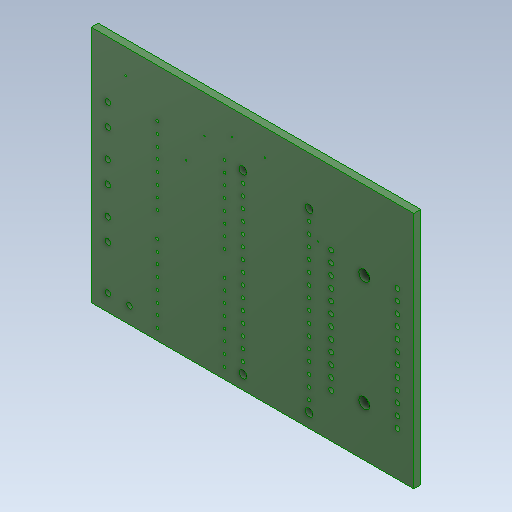
# Autodesk Inventor part: dog_driver_4.brd_Outline
Saved by Autodesk Inventor 2020 (Build 240168000, 168)
## iProperties
Created: 2019-07-14
Part Number: dog_driver_4.brd_Outline
Material: Generic
Document SubType Name: Modeling
Designer: psrob
Density: 1 g/cm^3
Appearance: Board Outline
Author: psrob
Autodesk Inventor part; units mm, degrees
ref_plane "YZ Plane" through (0, 0, 0) normal (1, 0, 0) x (0, 1, 0)
ref_plane "XZ Plane" through (0, 0, 0) normal (0, 1, 0) x (-1, 0, 0)
ref_plane "XY Plane" through (0, 0, 0) normal (0, 0, 1) x (1, 0, 0)
sketch "Sketch1" plane through (0, 0, 0) normal (0, 0, 1) x (1, 0, 0)
  line L0 (0, 0) -> (74.275, 0)
  line L1 (74.275, 0) -> (74.275, 54.915)
  line L2 (74.275, 54.915) -> (0, 54.915)
  line L3 (0, 54.915) -> (0, 0)
  circle A0 centre (50.16, 5.71) radius 0.4
  circle A1 centre (50.16, 8.26) radius 0.4
  circle A2 centre (50.16, 10.79) radius 0.4
  circle A3 centre (50.16, 13.34) radius 0.4
  circle A4 centre (50.16, 15.88) radius 0.4
  circle A5 centre (50.16, 18.41) radius 0.4
  circle A6 centre (50.16, 20.96) radius 0.4
  circle A7 centre (50.16, 23.5) radius 0.4
  circle A8 centre (50.16, 26.04) radius 0.4
  circle A9 centre (50.16, 28.58) radius 0.4
  circle A10 centre (50.16, 31.12) radius 0.4
  circle A11 centre (50.16, 33.66) radius 0.4
  circle A12 centre (50.16, 36.2) radius 0.4
  circle A13 centre (50.16, 38.73) radius 0.4
  circle A14 centre (50.16, 41.27) radius 0.4
  circle A15 centre (34.93, 41.27) radius 0.4
  circle A16 centre (34.93, 38.73) radius 0.4
  circle A17 centre (34.93, 36.2) radius 0.4
  circle A18 centre (34.93, 33.66) radius 0.4
  circle A19 centre (34.93, 31.12) radius 0.4
  circle A20 centre (34.93, 28.58) radius 0.4
  circle A21 centre (34.93, 26.04) radius 0.4
  circle A22 centre (34.93, 23.5) radius 0.4
  circle A23 centre (34.93, 20.96) radius 0.4
  circle A24 centre (34.93, 18.41) radius 0.4
  circle A25 centre (34.93, 15.88) radius 0.4
  circle A26 centre (34.93, 13.34) radius 0.4
  circle A27 centre (34.93, 10.79) radius 0.4
  circle A28 centre (34.93, 8.26) radius 0.4
  circle A29 centre (34.93, 5.71) radius 0.4
  circle A30 centre (3.81, 41.91) radius 0.65
  circle A31 centre (3.81, 36.91) radius 0.65
  circle A32 centre (3.81, 30.48) radius 0.65
  circle A33 centre (3.81, 25.48) radius 0.65
  circle A34 centre (3.81, 19.05) radius 0.65
  circle A35 centre (3.81, 14.05) radius 0.65
  circle A36 centre (3.81, 3.81) radius 0.65
  circle A37 centre (8.81, 3.81) radius 0.65
  circle A38 centre (15.24, 36.2) radius 0.3
  circle A39 centre (15.24, 33.66) radius 0.3
  circle A40 centre (30.73, 38.73) radius 0.3
  circle A41 centre (30.73, 41.27) radius 0.3
  circle A42 centre (15.24, 28.58) radius 0.3
  circle A43 centre (15.24, 31.12) radius 0.3
  circle A44 centre (30.73, 33.66) radius 0.3
  circle A45 centre (30.73, 31.12) radius 0.3
  circle A46 centre (15.24, 38.73) radius 0.3
  circle A47 centre (15.24, 26.04) radius 0.3
  circle A48 centre (30.73, 26.04) radius 0.3
  circle A49 centre (30.73, 43.82) radius 0.3
  circle A50 centre (30.73, 28.58) radius 0.3
  circle A51 centre (30.73, 36.2) radius 0.3
  circle A52 centre (15.24, 41.27) radius 0.3
  circle A53 centre (15.24, 43.82) radius 0.35
  circle A54 centre (15.24, 12.7) radius 0.3
  circle A55 centre (15.24, 10.16) radius 0.3
  circle A56 centre (30.73, 15.24) radius 0.3
  circle A57 centre (30.73, 17.78) radius 0.3
  circle A58 centre (15.24, 5.08) radius 0.3
  circle A59 centre (15.24, 7.62) radius 0.3
  circle A60 centre (30.73, 10.16) radius 0.3
  circle A61 centre (30.73, 7.62) radius 0.3
  circle A62 centre (15.24, 15.24) radius 0.3
  circle A63 centre (15.24, 2.54) radius 0.3
  circle A64 centre (30.73, 2.54) radius 0.3
  circle A65 centre (30.73, 20.32) radius 0.3
  circle A66 centre (30.73, 5.08) radius 0.3
  circle A67 centre (30.73, 12.7) radius 0.3
  circle A68 centre (15.24, 17.78) radius 0.3
  circle A69 centre (15.24, 20.32) radius 0.35
  circle A70 centre (55.25, 38.1) radius 0.555
  circle A71 centre (55.25, 35.56) radius 0.555
  circle A72 centre (55.25, 33.02) radius 0.555
  circle A73 centre (55.25, 30.48) radius 0.555
  circle A74 centre (55.25, 27.94) radius 0.555
  circle A75 centre (55.25, 25.4) radius 0.555
  circle A76 centre (55.25, 22.86) radius 0.555
  circle A77 centre (55.25, 20.32) radius 0.555
  circle A78 centre (55.25, 17.78) radius 0.555
  circle A79 centre (55.25, 15.24) radius 0.555
  circle A80 centre (55.25, 12.7) radius 0.555
  circle A81 centre (55.25, 10.16) radius 0.555
  circle A82 centre (70.48, 10.16) radius 0.555
  circle A83 centre (70.48, 12.7) radius 0.555
  circle A84 centre (70.48, 15.24) radius 0.555
  circle A85 centre (70.48, 17.78) radius 0.555
  circle A86 centre (70.48, 20.32) radius 0.555
  circle A87 centre (70.48, 22.86) radius 0.555
  circle A88 centre (70.48, 25.4) radius 0.555
  circle A89 centre (70.48, 27.94) radius 0.555
  circle A90 centre (70.48, 30.48) radius 0.555
  circle A91 centre (70.48, 33.02) radius 0.555
  circle A92 centre (70.48, 35.56) radius 0.555
  circle A93 centre (70.48, 38.1) radius 0.555
  circle A94 centre (62.87, 36.83) radius 1.27
  circle A95 centre (62.87, 11.43) radius 1.27
  circle A96 centre (50.165, 3.175) radius 0.889
  circle A97 centre (34.925, 3.175) radius 0.889
  circle A98 centre (34.925, 43.815) radius 0.889
  circle A99 centre (50.165, 43.815) radius 0.889
  circle A100 centre (52.1716, 38.3032) radius 0.175
  circle A101 centre (39.9542, 48.8696) radius 0.175
  circle A102 centre (7.9248, 49.1998) radius 0.175
  circle A103 centre (21.7932, 39.2938) radius 0.175
  circle A104 centre (32.3596, 49.1998) radius 0.175
  circle A105 centre (26.0858, 46.228) radius 0.175
  constraints: 106 centre point, 8 end point
extrude "dog_driver_4.brd_Outline" add sketch "Sketch1" along normal blind 1.6
body "Solid1"
